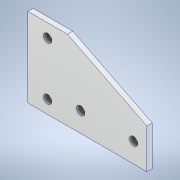
# Autodesk Inventor part: FrameJoint1515
Saved by Autodesk Inventor 2022.2 (Build 262287010, 287A)
## iProperties
Created: 2022-03-21
Part Number: FrameJoint1515
Material: アルミニウム 6061
Document SubType Name: Modeling
Designer: YusukeKunita
Density: 2.7 g/cm^3
Appearance: アルミニウム - フラット
Author: YusukeKunita
Autodesk Inventor part; units mm, degrees
ref_plane "YZ Plane" through (0, 0, 0) normal (1, 0, 0) x (0, 1, 0)
ref_plane "XZ Plane" through (0, 0, 0) normal (0, 1, 0) x (-1, 0, 0)
ref_plane "XY Plane" through (0, 0, 0) normal (0, 0, 1) x (1, 0, 0)
sketch "スケッチ1" plane through (0, 0, 0) normal (1, 0, 0) x (0, 1, 0)
  line L0 (0, 0) -> (45, 0)
  line L1 (45, 0) -> (45, 15)
  line L2 (45, 15) -> (0, 15) construction
  line L3 (0, 15) -> (0, 0)
  line L4 (0, 0) -> (15, 0)
  line L5 (15, 0) -> (15, 30) construction
  line L6 (15, 30) -> (0, 30)
  line L7 (0, 30) -> (0, 0)
  line L8 (15, 30) -> (45, 15)
  dimension "d0" = 15
  dimension "d1" = 15
  dimension "d2" = 30
  dimension "d3" = 30
  constraints: 18 end point, 4 parallel, 2 horizontal, 2 perpendicular
  measures "d0" distance of L0.end L1.end
  measures "d1" distance of L5.end L6.end
  measures "d2" distance between parallel lines of L5 L1
  measures "d3" distance of L4.end L5.end
extrude "押し出し1" add sketch "スケッチ1" along normal blind 2
sketch "スケッチ2" plane through (2, 0, 0) normal (1, 0, 0) x (0, 0, -1)
  line L0 (-30, 15) -> (-30, 0) projected
  line L1 (-30, 7.5) -> (0, 7.5) construction
  line L2 (0, 0) -> (0, 45) projected
  line L3 (0, 45) -> (-15, 45) projected
  line L4 (-7.5, 45) -> (-7.5, 0) construction
  line L5 (-30, 0) -> (0, 0) projected
  point P0 (-25, 7.5)
  point P1 (-5, 7.5)
  point P2 (-7.5, 20)
  point P3 (-7.5, 40)
  dimension "d6" = 20
  dimension "d7" = 5
  dimension "d8" = 20
  dimension "d9" = 5
  constraints: 6 point on line, 4 end point, 2 midpoint, 1 horizontal, 1 perpendicular
  measures "d6" distance of point (-7.5, 40) point (-7.5, 20)
  measures "d7" distance from line of L3 point (-7.5, 40)
  measures "d8" distance of point (-5, 7.5) point (-25, 7.5)
  measures "d9" distance from line of L0 point (-25, 7.5)
hole "穴1" at (2, 7.5, 25) at (2, 7.5, 5) at (2, 20, 7.5) at (2, 40, 7.5) direction (-1, 0, 0) diameter 3.2 end through all
